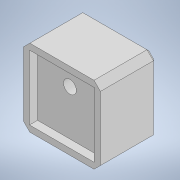
# Autodesk Inventor part: Idle Side Foot
Saved by Autodesk Inventor 2022 (Build 260153000, 153)
## iProperties
Created: 2022-05-29
Part Number: Idle Side Foot
Material: Generic
Document SubType Name: Modeling
Designer: Nick
Density: 1 g/cm^3
Appearance: Default
Author: Nick
Autodesk Inventor part; units mm, degrees
ref_plane "YZ Plane" through (0, 0, 0) normal (1, 0, 0) x (0, 1, 0)
ref_plane "XZ Plane" through (0, 0, 0) normal (0, 1, 0) x (-1, 0, 0)
ref_plane "XY Plane" through (0, 0, 0) normal (0, 0, 1) x (1, 0, 0)
sketch "Sketch1" plane through (0, 0, 0) normal (0, 0, 1) x (1, 0, 0)
  line L0 (0, 0) -> (24, 0)
  line L1 (24, 0) -> (24, 24)
  line L2 (24, 24) -> (0, 24)
  line L3 (0, 24) -> (0, 0)
  dimension "d0" = 24
  dimension "d1" = 24
  constraints: 8 end point, 2 parallel, 1 horizontal, 1 perpendicular
  measures "d0" distance of L2.end L1.end
  measures "d1" distance of L1.end L0.end
extrude "Extrusion1" add sketch "Sketch1" along normal blind 15
sketch "Sketch2" plane through (0, 0, 15) normal (0, 0, 1) x (1, 0, 0)
  line L0 (24, 0) -> (24, 24) projected
  line L1 (24, 24) -> (0, 24) projected
  line L2 (0, 24) -> (0, 0) projected
  line L3 (0, 0) -> (24, 0) projected
  line L4 (2, 22) -> (22, 22)
  line L5 (22, 22) -> (22, 2)
  line L6 (22, 2) -> (2, 2)
  line L7 (2, 2) -> (2, 22)
  dimension "d4" = 2
  constraints: 8 end point, 3 other
  measures "d4" distance between parallel lines of L1 L4
extrude "Extrusion2" add sketch "Sketch2" along normal blind 2.5
chamfer "Chamfer1" distance 2 angle 45 4 edges at (0, 24, 8.75) (0, 0, 8.75) (24, 0, 8.75) (24, 24, 8.75)
sketch "Sketch3" plane through (0, 0, 0) normal (0, 0, -1) x (-1, 0, 0)
  line L0 (-2, 22) -> (-2, 2) projected
  line L1 (-2, 2) -> (-22, 2) projected
  line L2 (-22, 2) -> (-22, 22) projected
  line L3 (-22, 22) -> (-2, 22) projected
  point P0 (0, 0)
  point P1 (-12, 16)
  point P2 (-12, 22)
  dimension "d10" = 6
  constraints: 1 midpoint, 1 vertical alignment
  measures "d10" distance from line of L3 point (-12, 16)
hole "Hole1" at (12, 16, 0) direction (0, 0, 1) diameter 4 depth 24 counterbore diameter 6.5 counterbore depth 10
chamfer "Chamfer2" distance 1 angle 45 8 edges at (12, 0, 0) (23, 1, 0) (24, 12, 0) (23, 23, 0) (12, 24, 0) (0, 12, 0) (1, 23, 0) (1, 1, 0)
thicken "Thicken1" operation add thickness 0.1 both sides no extend neighbours yes toward (1, 0, 0) faces at (22, 15.3333, 16.6667) (15.3333, 2, 16.6667) (2, 8.6667, 16.6667) (8.6667, 22, 15.8333)
chamfer "Chamfer3" distance 1.25 angle 45 1 edges at (12, 14, 10)
body "Solid1"
